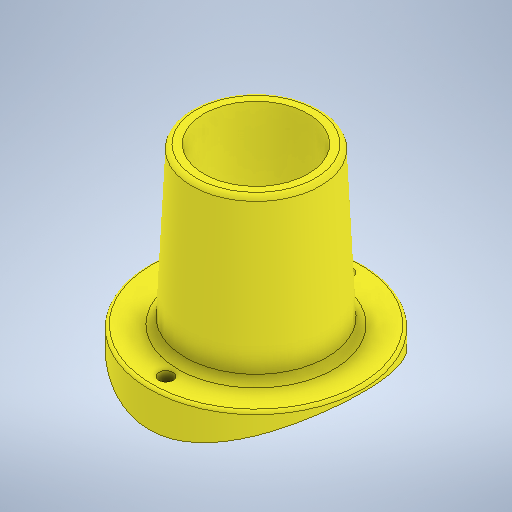
# Autodesk Inventor part: 131
Saved by Autodesk Inventor 2025.1 (Build 291241000, 241)
## iProperties
Created: 2024-08-01
Part Number: 131
Material: Aluminum 6061-AHC
Document SubType Name: Modeling
Designer: ffogue
Density: 2.7 g/cm^3
Appearance: Canary
Author: ffogue
Autodesk Inventor part; units mm, degrees
ref_plane "XZ Plane" through (0, 0, 0) normal (0, 1, 0) x (-1, 0, 0)
sketch "Sketch1" plane through (0, 0, 0) normal (0, 0, 1) x (1, 0, 0)
  circle A0 centre (0, 0) radius 22.5
  dimension "d0" = 45
  constraints: 1 centre point, 1 coincident
  measures "d0" diameter of A0
extrude "Extrusion1" add sketch "Sketch1" along normal blind 8
ref_plane "Work Plane1" through (0, 0, 0) normal (1, 0, 0) x (0, 1, 0)
sketch "Sketch3" plane through (0, 0, 0) normal (1, 0, 0) x (0, 1, 0)
  line L0 (22.5, 8) -> (-22.5, 8) projected
  line L1 (22.5, 0) -> (-22.5, 0) projected
  line L2 (0, 8) -> (0, 41)
  line L3 (0, 41) -> (-13.5, 41)
  line L4 (-13.5, 41) -> (-15, 8)
  point P0 (0, 0)
  dimension "d4" = 27
  dimension "d5" = 33
  dimension "d6" = 30
  constraints: 6 end point, 1 midpoint, 1 perpendicular, 1 point on line, 1 vertical
  measures "d4" diameter of L3.end L2
  measures "d5" distance between parallel lines of L0 L3
  measures "d6" diameter of L4.end L2
revolve "Revolution1" add sketch "Sketch3" angle 360 about axis through (0, 0, 8) along (0, 0, 1)
fillet "Fillet1" radius 1.5 1 edges at (0, 15, 8)
sketch "Sketch5" plane through (0, 0, 0) normal (1, 0, 0) x (0, 1, 0)
  arc A0 (22.5, 0) -> (-22.5, 0) centre (0, -33.6749) ccw
  line L0 (22.5, 0) -> (-22.5, 0) projected
  point P0 (0, 0)
  dimension "d16" = 81
  constraints: 2 end point, 2 point on circle, 1 centre point
  measures "d16" diameter of A0
extrude "Extrusion2" cut sketch "Sketch5" along normal mid plane 45
fillet "Fillet2" radius 0.6 1 edges at (-22.5, 0, 8)
fillet "Fillet3" radius 1 1 edges at (0, 13.5, 41)
sketch "Sketch6" plane through (0, 0, 41) normal (0, 0, 1) x (1, 0, 0)
  circle A0 centre (0, 0) radius 13.5 projected
  constraints: 1 coincident
hole "Hole2" at (0, 0, 41) direction (0, 0, -1) diameter 20 end through all counterbore diameter 22 counterbore depth 27
sketch "Sketch7" plane through (0, 0, 8) normal (0, 0, 1) x (1, 0, 0)
  point P0 (0, 0)
  point P1 (0, -19)
  point P2 (0, 19)
  dimension "d27" = 19
  dimension "d28" = 19
  constraints: 2 vertical alignment
  measures "d27" distance of point (0, 0) point (0, -19)
  measures "d28" distance of point (0, 19) point (0, 0)
hole "Hole3" at (0, -19, 8) at (0, 19, 8) direction (0, 0, -1) diameter 3 end through all
ref_plane "Work Plane2" through (0, 0, 0) normal (0, 0, 1) x (1, 0, 0)
sketch "Sketch9" plane through (0, 0, 0) normal (0, 0, 1) x (1, 0, 0)
  circle A0 centre (0, 0) radius 22.5
  dimension "d39" = 45
  constraints: 1 centre point, 1 coincident
  measures "d39" diameter of A0
equation "\"d28\" = d27"
body "Solid1"
